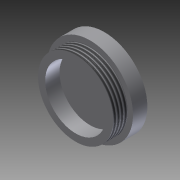
# Autodesk Inventor part: cap_a
Saved by Autodesk Inventor 2011 (Build 150239000, 239)
## iProperties
Created: 2011-01-25
Part Number: cap_a
Document SubType Name: Modeling
Designer: labuser
Density: 1 g/cm^3
Author: labuser
Autodesk Inventor part; units mm, degrees
ref_plane "YZ Plane" through (0, 0, 0) normal (1, 0, 0) x (0, 1, 0)
ref_plane "XZ Plane" through (0, 0, 0) normal (0, 1, 0) x (-1, 0, 0)
ref_plane "XY Plane" through (0, 0, 0) normal (0, 0, 1) x (1, 0, 0)
sketch "Sketch1" plane through (0, 0, 0) normal (0, 0, 1) x (1, 0, 0)
  circle A0 centre (0, 0) radius 7.62
  dimension "d0" = 15.24
  constraints: 1 centre point, 1 coincident
  measures "d0" diameter of A0
extrude "Extrusion1" add sketch "Sketch1" along normal blind 2.54
sketch "Sketch2" plane through (0, 0, 2.54) normal (0, 0, 1) x (1, 0, 0)
  circle A0 centre (0, 0) radius 7.62 projected
  circle A1 centre (0, 0) radius 6.6675
  dimension "d3" = 13.335
  constraints: 1 centre point, 1 coincident
  measures "d3" diameter of A1
extrude "Extrusion2" add sketch "Sketch2" along normal blind 2.54 contours A1
thread "Thread1" size "4-40 UNC" class "2A" standard "ANSI Unified Screw Threads" full length
sketch "Sketch3" plane through (0, 0, 5.08) normal (0, 0, 1) x (1, 0, 0)
  circle A0 centre (0, 0) radius 6.6675 projected
  circle A1 centre (0, 0) radius 5.3975
  dimension "d8" = 10.795
  constraints: 1 centre point, 1 coincident
  measures "d8" diameter of A1
extrude "Extrusion3" cut sketch "Sketch3" against normal blind 2.54 contours A1
body "Solid1"
